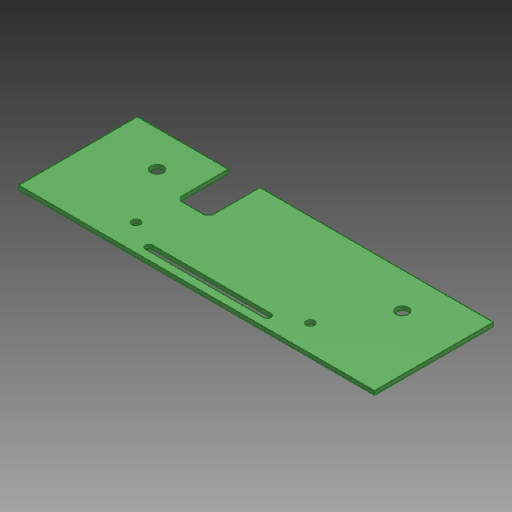
# Autodesk Inventor part: Ballsensorplatine
Saved by Autodesk Inventor 2019.4 (Build 234330000, 330)
## iProperties
Part Number: Ballsensorplatine
Material: Phenolharz
Document SubType Name: Modeling
Designer: rYan
Density: 1.38 g/cm^3
Appearance: Glatt - waldgrün
Mass: 3.47544 g
Surface Area: 54.0002 cm^2
Volume: 2.51843 cm^3
Author: rYan
Autodesk Inventor part; units mm, degrees
ref_plane "YZ Plane" through (0, 0, 0) normal (1, 0, 0) x (0, 1, 0)
ref_plane "XZ Plane" through (0, 0, 0) normal (0, 1, 0) x (-1, 0, 0)
ref_plane "XY Plane" through (0, 0, 0) normal (0, 0, 1) x (1, 0, 0)
sketch "Skizze1" plane through (0, 0, 0) normal (0, 0, 1) x (1, 0, 0)
  line L0 (-45, 15) -> (45, 15)
  line L1 (45, 15) -> (45, -15)
  line L2 (45, -15) -> (-45, -15)
  line L3 (-45, -15) -> (-45, 15)
  line L4 (-45, 15) -> (45, -15) construction
  line L5 (45, 15) -> (-45, -15) construction
  point P0 (0, 0)
  dimension "d0" = 30
  dimension "d1" = 90
  constraints: 12 end point, 2 midpoint, 2 parallel, 1 horizontal, 1 perpendicular
  measures "d0" distance of L0.end L1.end
  measures "d1" distance of L0.start L0.end
extrude "Extrusion1" add sketch "Skizze1" along normal blind 1
sketch "Skizze4" plane through (0, 0, 1) normal (0, 0, 1) x (1, 0, 0)
  line L0 (15, -12.1) -> (-15, -12.1) construction
  line L1 (15, -11.2) -> (-15, -11.2)
  line L2 (-15, -13) -> (15, -13)
  arc A0 (15, -13) -> (15, -11.2) centre (15, -12.1) ccw
  arc A1 (-15, -11.2) -> (-15, -13) centre (-15, -12.1) ccw
  line L3 (0, 21) -> (0, -21) projected
  line L4 (-45, -15) -> (45, -15) projected
  point P0 (0, 0)
  point P1 (0, -12.1)
  dimension "d25" = 1.8
  dimension "d26" = 30
  dimension "d27" = 2
  constraints: 8 end point, 4 point on circle, 4 tangent, 2 centre point, 1 horizontal, 1 midpoint, 1 parallel, 1 other
  measures "d25" diameter of A1
  measures "d26" distance of L0.start L0.end
  measures "d27" distance between parallel lines of L4 L2
extrude "Extrusion2" cut sketch "Skizze4" against normal through all
sketch "Skizze2" plane through (0, 0, 1) normal (0, 0, 1) x (1, 0, 0)
  line L0 (31, 6) -> (-31, 6) construction
  line L1 (45, 15) -> (-45, 15) projected
  line L2 (0, 21) -> (0, -21) projected
  line L3 (-45, -15) -> (45, -15) projected
  dimension "d5" = 62
  dimension "d48" = 21
  constraints: 2 coincident, 2 end point, 1 symmetric about line
  measures "d5" distance of L0.start L0.end
  measures "d48" distance between parallel lines of L0 L3
hole "Bohrung1" at (-31, 6, 1) at (31, 6, 1) direction (0, 0, -1) diameter 3.1 end through all
sketch "Skizze5" plane through (0, 0, 1) normal (0, 0, 1) x (1, 0, 0)
  line L0 (-45, -15) -> (45, -15) projected
  line L1 (0, 21) -> (0, -21) projected
  point P0 (0, 0)
  point P1 (22.05, -8.3)
  point P2 (-22.05, -8.3)
  dimension "d30" = 6.7
  dimension "d31" = 44.1
  constraints: 1 symmetric about line
  measures "d30" distance from line of L0 point (22.05, -8.3)
  measures "d31" distance of point (-22.05, -8.3) point (22.05, -8.3)
hole "Bohrung3" at (22.05, -8.3, 1) at (-22.05, -8.3, 1) direction (0, 0, -1) diameter 2.1 end through all
sketch "Skizze7" plane through (0, 0, 1) normal (0, 0, 1) x (1, 0, 0)
  line L0 (0, 21) -> (0, -21) projected
  line L1 (-45, -15) -> (45, -15) projected
  line L2 (-22, 15) -> (-14, 15)
  line L3 (-14, 15) -> (-14, 2)
  line L4 (-14, 2) -> (-22, 2)
  line L5 (-22, 2) -> (-22, 15)
  line L6 (-18, 2) -> (-18, 15) construction
  line L7 (45, 15) -> (-45, 15) construction
  point P0 (0, 0)
  dimension "d49" = 18
  dimension "d50" = 17
  dimension "d51" = 8
  constraints: 10 end point, 2 midpoint, 2 parallel, 1 collinear, 1 horizontal, 1 perpendicular
  measures "d49" distance between parallel lines of L0 L6
  measures "d50" distance between parallel lines of L1 L4
  measures "d51" distance between parallel lines of L3 L5
extrude "Extrusion4" cut sketch "Skizze7" against normal through all
chamfer "Fase1" distance 1 angle 45 2 edges at (-22, 2, 0.5) (-14, 2, 0.5)
